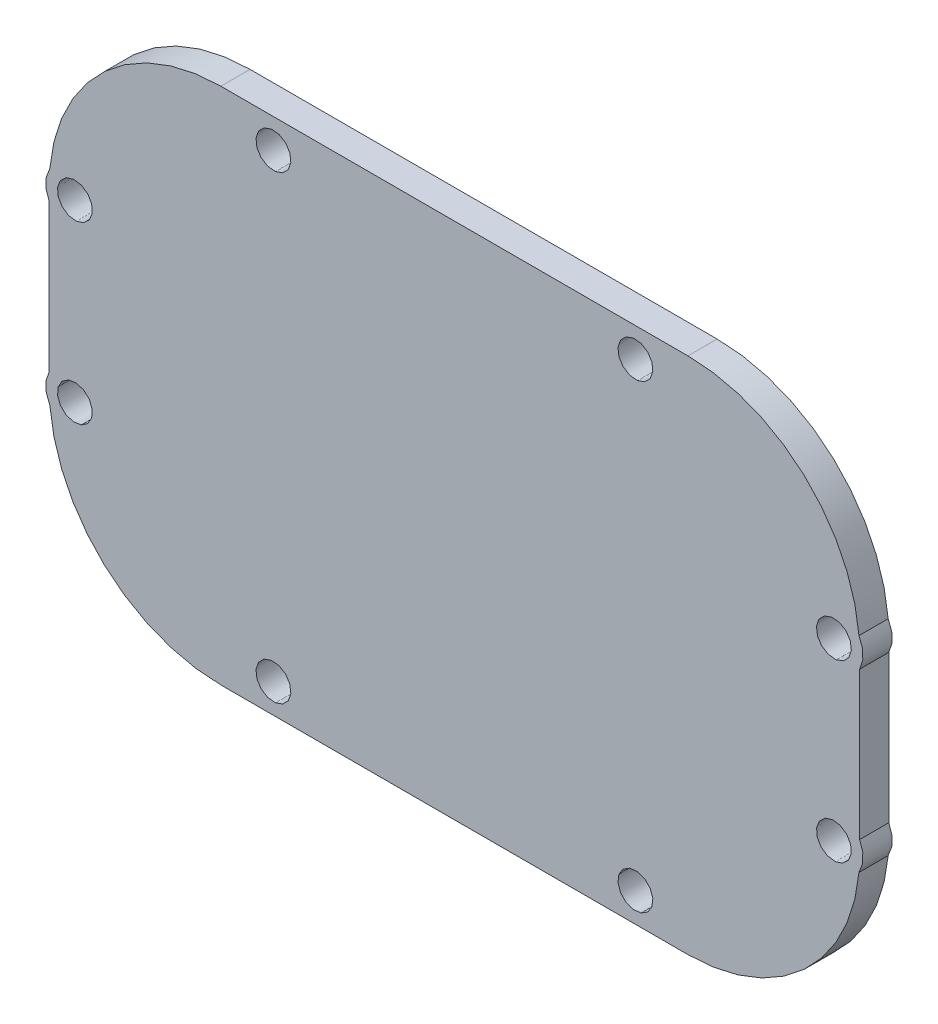
# Autodesk Inventor part: front_acryl
Saved by Autodesk Inventor 2024 (Build 280153000, 153)
## iProperties
Created: 2026-08-20
Part Number: front_acryl
Material: Generic
Document SubType Name: Modeling
Designer: schar
Density: 1 g/cm^3
Appearance: Default
Author: schar
Autodesk Inventor part; units mm, degrees
ref_plane "YZ Plane" through (0, 0, 0) normal (1, 0, 0) x (0, 1, 0)
ref_plane "XZ Plane" through (0, 0, 0) normal (0, 1, 0) x (-1, 0, 0)
ref_plane "XY Plane" through (0, 0, 0) normal (0, 0, 1) x (1, 0, 0)
sketch "Sketch1" plane through (0, 0, 0) normal (0, 0, 1) x (1, 0, 0)
  line L0 (-32.7, -6.0134) -> (-32.7, 6.0134) projected
  arc A0 (-32.6116, 8.9958) -> (-32.7, 6.0134) centre (-32.5, 7.5) ccw projected
  arc A1 (-20, 20.2) -> (-32.6116, 8.9958) centre (-20, 7.5) ccw projected
  line L1 (-20, 20.2) -> (-16.9142, 20.2) projected
  arc A2 (-14.0858, 20.2) -> (-16.9142, 20.2) centre (-15.5, 19.7) ccw projected
  line L2 (-14.0858, 20.2) -> (14.0858, 20.2) projected
  arc A3 (16.9142, 20.2) -> (14.0858, 20.2) centre (15.5, 19.7) ccw projected
  line L3 (16.9142, 20.2) -> (20, 20.2) projected
  arc A4 (32.6116, 8.9958) -> (20, 20.2) centre (20, 7.5) ccw projected
  arc A5 (32.7, 6.0134) -> (32.6116, 8.9958) centre (32.5, 7.5) ccw projected
  line L4 (32.7, 6.0134) -> (32.7, -6.0134) projected
  arc A6 (32.6116, -8.9958) -> (32.7, -6.0134) centre (32.5, -7.5) ccw projected
  arc A7 (20, -20.2) -> (32.6116, -8.9958) centre (20, -7.5) ccw projected
  line L5 (20, -20.2) -> (16.9142, -20.2) projected
  arc A8 (14.0858, -20.2) -> (16.9142, -20.2) centre (15.5, -19.7) ccw projected
  line L6 (14.0858, -20.2) -> (-14.0858, -20.2) projected
  arc A9 (-16.9142, -20.2) -> (-14.0858, -20.2) centre (-15.5, -19.7) ccw projected
  line L7 (-16.9142, -20.2) -> (-20, -20.2) projected
  arc A10 (-32.6116, -8.9958) -> (-20, -20.2) centre (-20, -7.5) ccw projected
  arc A11 (-32.7, -6.0134) -> (-32.6116, -8.9958) centre (-32.5, -7.5) ccw projected
  arc A12 (34.6474, -8.7801) -> (34.7032, -6.3185) centre (32.5, -7.5) ccw projected
  line L8 (34.7032, -6.3185) -> (34.7032, 6.3185) projected
  arc A13 (34.7032, 6.3185) -> (34.6474, 8.7801) centre (32.5, 7.5) ccw projected
  arc A14 (34.6474, 8.7801) -> (20, 22.2032) centre (20, 7.5) ccw projected
  line L9 (20, 22.2032) -> (-20, 22.2032) projected
  arc A15 (-20, 22.2032) -> (-34.6474, 8.7801) centre (-20, 7.5) ccw projected
  arc A16 (-34.6474, 8.7801) -> (-34.7032, 6.3185) centre (-32.5, 7.5) ccw projected
  line L10 (-34.7032, 6.3185) -> (-34.7032, -6.3185) projected
  arc A17 (-34.7032, -6.3185) -> (-34.6474, -8.7801) centre (-32.5, -7.5) ccw projected
  arc A18 (-34.6474, -8.7801) -> (-20, -22.2032) centre (-20, -7.5) ccw projected
  line L11 (-20, -22.2032) -> (20, -22.2032) projected
  arc A19 (20, -22.2032) -> (34.6474, -8.7801) centre (20, -7.5) ccw projected
  arc A20 (-31.6356, 8.7259) -> (-32.6116, 8.9958) centre (-32.5, 7.5) ccw projected
  arc A21 (-20, 19.2) -> (-31.6356, 8.7259) centre (-20, 7.5) ccw projected
  line L12 (-16.9142, 19.2) -> (-20, 19.2) projected
  arc A22 (-16.9142, 20.2) -> (-16.9142, 19.2) centre (-15.5, 19.7) ccw projected
  line L13 (-20, 20.2) -> (-16.9142, 20.2) projected
  arc A23 (-20, 20.2) -> (-32.6116, 8.9958) centre (-20, 7.5) ccw projected
  arc A24 (-32.7, 6.0134) -> (-31.7, 6.2311) centre (-32.5, 7.5) ccw projected
  line L14 (-32.7, -6.0134) -> (-32.7, 6.0134) projected
  arc A25 (-31.7, -6.2311) -> (-32.7, -6.0134) centre (-32.5, -7.5) ccw projected
  line L15 (-31.7, 6.2311) -> (-31.7, -6.2311) projected
  line L16 (-31.7, 6.2311) -> (-31.7, -6.2311) projected
  arc A26 (-31.6356, -8.7259) -> (-31.7, -6.2311) centre (-32.5, -7.5) ccw projected
  arc A27 (-31.6356, -8.7259) -> (-20, -19.2) centre (-20, -7.5) ccw projected
  line L17 (-20, -19.2) -> (-16.9142, -19.2) projected
  arc A28 (-14.0858, -19.2) -> (-16.9142, -19.2) centre (-15.5, -19.7) ccw projected
  line L18 (-14.0858, -19.2) -> (14.0858, -19.2) projected
  arc A29 (16.9142, -19.2) -> (14.0858, -19.2) centre (15.5, -19.7) ccw projected
  line L19 (16.9142, -19.2) -> (20, -19.2) projected
  arc A30 (20, -19.2) -> (31.6356, -8.7259) centre (20, -7.5) ccw projected
  arc A31 (31.7, -6.2311) -> (31.6356, -8.7259) centre (32.5, -7.5) ccw projected
  line L20 (31.7, -6.2311) -> (31.7, 6.2311) projected
  arc A32 (31.6356, 8.7259) -> (31.7, 6.2311) centre (32.5, 7.5) ccw projected
  arc A33 (31.6356, 8.7259) -> (20, 19.2) centre (20, 7.5) ccw projected
  line L21 (20, 19.2) -> (16.9142, 19.2) projected
  arc A34 (14.0858, 19.2) -> (16.9142, 19.2) centre (15.5, 19.7) ccw projected
  line L22 (14.0858, 19.2) -> (-14.0858, 19.2) projected
  arc A35 (-16.9142, 19.2) -> (-14.0858, 19.2) centre (-15.5, 19.7) ccw projected
  line L23 (-16.9142, 19.2) -> (-20, 19.2) projected
  arc A36 (-20, 19.2) -> (-31.6356, 8.7259) centre (-20, 7.5) ccw projected
  arc A37 (-31.7, 6.2311) -> (-31.6356, 8.7259) centre (-32.5, 7.5) ccw projected
  line L24 (-30.1616, -8.3842) -> (-30.2, -6.5202) projected
  line L25 (-30.2, -6.5202) -> (-30.2, 6.5202) projected
  line L26 (-30.2, 6.5202) -> (-30.1616, 8.3842) projected
  arc A38 (-20, 17.7) -> (-30.1616, 8.3842) centre (-20, 7.5) ccw projected
  line L27 (-20, 17.7) -> (20, 17.7) projected
  arc A39 (30.1616, 8.3842) -> (20, 17.7) centre (20, 7.5) ccw projected
  line L28 (30.1616, 8.3842) -> (30.2, 6.5202) projected
  line L29 (30.2, 6.5202) -> (30.2, -6.5202) projected
  line L30 (30.2, -6.5202) -> (30.1616, -8.3842) projected
  arc A40 (20, -17.7) -> (30.1616, -8.3842) centre (20, -7.5) ccw projected
  line L31 (20, -17.7) -> (-20, -17.7) projected
  arc A41 (-30.1616, -8.3842) -> (-20, -17.7) centre (-20, -7.5) ccw projected
  arc A42 (-14.0858, -20.2) -> (-14.0858, -19.2) centre (-15.5, -19.7) ccw projected
  line L32 (14.0858, -20.2) -> (-14.0858, -20.2) projected
  arc A43 (14.0858, -19.2) -> (14.0858, -20.2) centre (15.5, -19.7) ccw projected
  line L33 (-14.0858, -19.2) -> (14.0858, -19.2) projected
  arc A44 (-16.9142, -19.2) -> (-16.9142, -20.2) centre (-15.5, -19.7) ccw projected
  line L34 (-20, -19.2) -> (-16.9142, -19.2) projected
  arc A45 (-31.6356, -8.7259) -> (-20, -19.2) centre (-20, -7.5) ccw projected
  arc A46 (-32.6116, -8.9958) -> (-31.6356, -8.7259) centre (-32.5, -7.5) ccw projected
  arc A47 (-32.6116, -8.9958) -> (-20, -20.2) centre (-20, -7.5) ccw projected
  line L35 (-16.9142, -20.2) -> (-20, -20.2) projected
  arc A48 (31.6356, -8.7259) -> (32.6116, -8.9958) centre (32.5, -7.5) ccw projected
  arc A49 (20, -19.2) -> (31.6356, -8.7259) centre (20, -7.5) ccw projected
  line L36 (16.9142, -19.2) -> (20, -19.2) projected
  arc A50 (16.9142, -20.2) -> (16.9142, -19.2) centre (15.5, -19.7) ccw projected
  line L37 (20, -20.2) -> (16.9142, -20.2) projected
  arc A51 (20, -20.2) -> (32.6116, -8.9958) centre (20, -7.5) ccw projected
  arc A52 (-14.0858, -20.2) -> (-14.0858, -19.2) centre (-15.5, -19.7) ccw projected
  line L38 (14.0858, -20.2) -> (-14.0858, -20.2) projected
  arc A53 (14.0858, -19.2) -> (14.0858, -20.2) centre (15.5, -19.7) ccw projected
  line L39 (-14.0858, -19.2) -> (14.0858, -19.2) projected
  arc A54 (32.7, -6.0134) -> (31.7, -6.2311) centre (32.5, -7.5) ccw projected
  line L40 (32.7, 6.0134) -> (32.7, -6.0134) projected
  arc A55 (31.7, 6.2311) -> (32.7, 6.0134) centre (32.5, 7.5) ccw projected
  line L41 (31.7, -6.2311) -> (31.7, 6.2311) projected
  arc A56 (16.9142, 19.2) -> (16.9142, 20.2) centre (15.5, 19.7) ccw projected
  line L42 (20, 19.2) -> (16.9142, 19.2) projected
  arc A57 (31.6356, 8.7259) -> (20, 19.2) centre (20, 7.5) ccw projected
  arc A58 (32.6116, 8.9958) -> (31.6356, 8.7259) centre (32.5, 7.5) ccw projected
  arc A59 (32.6116, 8.9958) -> (20, 20.2) centre (20, 7.5) ccw projected
  line L43 (16.9142, 20.2) -> (20, 20.2) projected
  arc A60 (14.0858, 20.2) -> (14.0858, 19.2) centre (15.5, 19.7) ccw projected
  line L44 (-14.0858, 20.2) -> (14.0858, 20.2) projected
  arc A61 (-14.0858, 19.2) -> (-14.0858, 20.2) centre (-15.5, 19.7) ccw projected
  line L45 (14.0858, 19.2) -> (-14.0858, 19.2) projected
  point P0 (0, 0)
extrude "Extrusion1" add sketch "Sketch1" along normal blind 2.5 contours L0 A24 L15 A25 | A46 A27 L17 A44 L7 A10 | L15 A37 A21 L12 A35 L22 A34 L21 A33 A32 L20 A31 A30 L19 A29 L18 A28 L17 A27 A26 | A1 L1 A22 L12 A21 A20 | A42 L18 A43 L6 | L2 A60 L22 A61 | A50 L19 A30 A48 A7 L5 | L3 A4 A58 A33 L21 A56 | A54 L20 A55 L4 | A19 L11 A18 A17 L10 A16 A15 L9 A14 A13 L8 A12 | L24 L25 L26 A38 L27 A39 L28 L29 L30 A40 L31 A41
body "Solid1"
